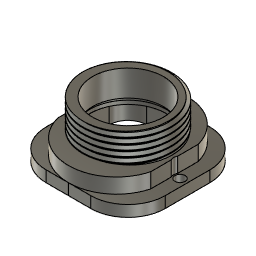
camera_holder_v10 (Autodesk Fusion 360 design; units mm, degrees)
Autodesk Fusion 360 part; units mm, degrees
sketch "Sketch1" plane through (0, 0, 0) normal (0, 0, 1) x (1, 0, 0)
  circle A0 centre (0, 0) radius 8
  circle A1 centre (14, 0) radius 1.375
  circle A2 centre (-14, 0) radius 1.375
  line L0 (-6.0043, 11.0001) -> (5.9948, 10.9999)
  line L1 (6, -16) -> (-6, -16)
  arc A3 (-16, -6) -> (-6, -16) centre (-6, -6) ccw
  line L2 (-16, -6) -> (-16, 6)
  arc A4 (-6, 16) -> (-16, 6) centre (-6, 6) ccw
  line L3 (-6, 16) -> (6, 16)
  arc A5 (16, 6) -> (6, 16) centre (6, 6) ccw
  line L4 (16, 6) -> (16, -6)
  arc A6 (6, -16) -> (16, -6) centre (6, -6) ccw
  line L5 (-11.0201, -5.8284) -> (-11.0201, 5.9457)
  line L6 (10.9799, 6.0014) -> (10.9799, -5.8832)
  line L7 (5.9985, -11.0001) -> (-5.9208, -10.9999)
  line L8 (-12.5201, -6.3696) -> (-12.5201, 6.4183)
  line L9 (12.4799, 6.418) -> (12.4799, -6.3695)
  line L10 (13.5, 2) -> (13.5, -2) construction
  arc A7 (-6.0043, 11.0001) -> (-11.0201, 5.9457) centre (-5.9656, 5.9457) ccw
  arc A8 (10.9799, 6.0014) -> (5.9948, 10.9999) centre (5.9947, 6.0147) ccw
  arc A9 (5.9985, -11.0001) -> (10.9799, -5.8832) centre (5.8611, -5.8832) ccw
  arc A10 (-11.0201, -5.8284) -> (-5.9208, -10.9999) centre (-5.9208, -5.9001) ccw
  arc A11 (12.4799, 6.418) -> (-12.5201, 6.4183) centre (-0.0201, 3.0556) ccw
  arc A12 (-12.5201, -6.3696) -> (12.4799, -6.3695) centre (-0.0201, -3.0725) ccw
  circle A13 centre (0, 0) radius 10.25
  dimension "d5" = 16
  dimension "d6" = 2.75
  dimension "d33" = 2.75
  dimension "d35" = 22
  dimension "d37" = 22
  dimension "d39" = 11
  dimension "d40" = 11
  dimension "d41" = 20.5
  constraint coincident A0.centre A13.centre
  constraint tangent L1 A6
  constraint tangent A4 L3
  constraint tangent L1 A3
  constraint tangent A5 L4
  constraint tangent A3 L2
  constraint tangent L4 A6
  constraint tangent L2 A4
  constraint tangent L3 A5
  constraint perpendicular L0 L10
  constraint tangent L5 A7
  constraint tangent L0 A8
  constraint tangent L6 A9
  constraint tangent L7 A10
  constraint concentric A0 A13
  measures "d5" diameter of A0
  measures "d6" diameter of A1
  measures "d33" diameter of A2
  measures "d35" distance of L0 L7
  measures "d37" distance of L5 L6
  measures "d39" distance of A0.centre L7
  measures "d40" distance of A0.centre L0
  measures "d41" diameter of A13
extrude "Extrude1" add sketch "Sketch1" along normal blind 3 contours L1 L3 A5 L4 A6 L9 A11 A12 | L1 A3 L2 A4 L3 L8 A11 A12 | L8 L9 A11 A12 makes body 1
extrude "Extrude2" add sketch "Sketch1" along normal blind 7 contours A0 | L0 L5 L6 L7 A7 A8 A9 A10 | A13 bodies 1
extrude "Extrude3" cut sketch "Sketch1" along normal blind 6 contours L0 L5 L6 L7 A7 A8 A9 A10 | A13 bodies 1 makes body 2 at (-2.0148, -0.2372, 7)
extrude "Extrude4" cut sketch "Sketch1" along normal blind 20 contours A0 bodies 1 2
sketch "Sketch2" plane through (0, 0, 0) normal (0, 0, 1) x (1, 0, 0)
  circle A0 centre (0, 0) radius 11.1125
  constraint coincident A0.centre origin
extrude "Extrude5" add sketch "Sketch2" along normal blind 8 separate body makes body 3
move_body "Move1" bodies 3 to x (1, 0, 0) y (0, 1, 0) z (0, 0, 1) at (0, 0, 7)
hole "Hole1" at (0, 0, 15) direction (0, 0, -1) diameter 19 depth 29 tip angle 118 bodies 3
extrude "Extrude6" add sketch "Sketch1" along normal blind 7 contours L8 L9 A11 A12 bodies 1 2
hole "Hole2" at (14, 0, 7) direction (0, 0, -1) diameter 3.5 depth 4 tip angle 180 bodies 1
sketch "Sketch3" plane through (0, 0, 0) normal (0, 0, 1) x (1, 0, 0)
  line L0 (0, 19) -> (0, -19) construction
hole "Hole3" at (-14, 0, 7) direction (0, 0, -1) diameter 3.5 depth 4 tip angle 180 bodies 1
thread "Thread3" "ISO Metric profile 24.0 M24x1.5 6g" major diameter 23.85 minor diameter 22.1319 pitch 1.5 angle 60 modelled right hand crest width 0.2123 on face at (11.0573, -1.1064, 12.3333) crest through (11.925, 0, 6.625) on bodies 3
extrude "Extrude7" cut sketch "Sketch1" along normal blind 8 contours A13 bodies 1 3
